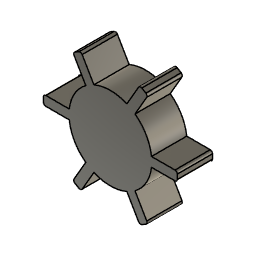
Waterwheel_6 (Autodesk Fusion 360 design; units mm, degrees)
Autodesk Fusion 360 part; units mm, degrees
sketch "スケッチ1" plane through (0, 0, 0) normal (0, 1, 0) x (-1, 0, 0)
  line L0 (-1750, 200) -> (-2750, 200)
  line L1 (-2850, 100) -> (-2850, -100)
  line L2 (-2750, -200) -> (-1750, -200)
  line L3 (-1750, 200) -> (0, 200) construction
  line L4 (0, 200) -> (0, -200) construction
  line L5 (0, -200) -> (-1750, -200) construction
  arc A0 (-2750, 200) -> (-2850, 100) centre (-2750, 100) ccw
  arc A1 (-2850, -100) -> (-2750, -200) centre (-2750, -100) ccw
  line L6 (-173.2051, 100) -> (173.2051, -100) construction
  arc A2 (-1548.2051, -2281.5699) -> (-1511.6025, -2418.1724) centre (-1461.6025, -2331.5699) ccw
  line L7 (-1201.7949, -2481.5699) -> (-701.7949, -1615.5445)
  line L8 (-1048.2051, -1415.5445) -> (-1548.2051, -2281.5699)
  arc A3 (-1338.3975, -2518.1724) -> (-1201.7949, -2481.5699) centre (-1288.3975, -2431.5699) ccw
  line L9 (-1048.2051, -1415.5445) -> (-173.2051, 100) construction
  line L10 (173.2051, -100) -> (-701.7949, -1615.5445) construction
  line L11 (-1511.6025, -2418.1724) -> (-1338.3975, -2518.1724)
  line L12 (-173.2051, -100) -> (173.2051, 100) construction
  arc A4 (1201.7949, -2481.5699) -> (1338.3975, -2518.1724) centre (1288.3975, -2431.5699) ccw
  line L13 (1548.2051, -2281.5699) -> (1048.2051, -1415.5445)
  line L14 (701.7949, -1615.5445) -> (1201.7949, -2481.5699)
  arc A5 (1511.6025, -2418.1724) -> (1548.2051, -2281.5699) centre (1461.6025, -2331.5699) ccw
  line L15 (701.7949, -1615.5445) -> (-173.2051, -100) construction
  line L16 (173.2051, 100) -> (1048.2051, -1415.5445) construction
  line L17 (1338.3975, -2518.1724) -> (1511.6025, -2418.1724)
  line L18 (0, -200) -> (0, 200) construction
  arc A6 (2750, -200) -> (2850, -100) centre (2750, -100) ccw
  line L19 (2750, 200) -> (1750, 200)
  line L20 (1750, -200) -> (2750, -200)
  arc A7 (2850, 100) -> (2750, 200) centre (2750, 100) ccw
  line L21 (1750, -200) -> (0, -200) construction
  line L22 (0, 200) -> (1750, 200) construction
  line L23 (2850, -100) -> (2850, 100)
  line L24 (173.2051, -100) -> (-173.2051, 100) construction
  arc A8 (1548.2051, 2281.5699) -> (1511.6025, 2418.1724) centre (1461.6025, 2331.5699) ccw
  line L25 (1201.7949, 2481.5699) -> (701.7949, 1615.5445)
  line L26 (1048.2051, 1415.5445) -> (1548.2051, 2281.5699)
  arc A9 (1338.3975, 2518.1724) -> (1201.7949, 2481.5699) centre (1288.3975, 2431.5699) ccw
  line L27 (1048.2051, 1415.5445) -> (173.2051, -100) construction
  line L28 (-173.2051, 100) -> (701.7949, 1615.5445) construction
  line L29 (1511.6025, 2418.1724) -> (1338.3975, 2518.1724)
  line L30 (173.2051, 100) -> (-173.2051, -100) construction
  arc A10 (-1201.7949, 2481.5699) -> (-1338.3975, 2518.1724) centre (-1288.3975, 2431.5699) ccw
  line L31 (-1548.2051, 2281.5699) -> (-1048.2051, 1415.5445)
  line L32 (-701.7949, 1615.5445) -> (-1201.7949, 2481.5699)
  arc A11 (-1511.6025, 2418.1724) -> (-1548.2051, 2281.5699) centre (-1461.6025, 2331.5699) ccw
  line L33 (-701.7949, 1615.5445) -> (173.2051, 100) construction
  line L34 (-173.2051, -100) -> (-1048.2051, 1415.5445) construction
  line L35 (-1338.3975, 2518.1724) -> (-1511.6025, 2418.1724)
  arc A12 (-1048.2051, 1415.5445) -> (-1750, 200) centre (0, 0) ccw
  arc A13 (701.7949, 1615.5445) -> (-701.7949, 1615.5445) centre (0, 0) ccw
  arc A14 (1750, 200) -> (1048.2051, 1415.5445) centre (0, 0) ccw
  arc A15 (1048.2051, -1415.5445) -> (1750, -200) centre (0, 0) ccw
  arc A16 (-1750, -200) -> (-1048.2051, -1415.5445) centre (0, 0) ccw
  arc A17 (-701.7949, -1615.5445) -> (701.7949, -1615.5445) centre (0, 0) ccw
  dimension "d19" = 100
  dimension "d20" = 400
  dimension "d21" = 1000
  dimension "d22" = 1750
  dimension "d24" = 360
  constraint coincident A12.centre A13.centre
  constraint horizontal L0
  constraint vertical L1
  constraint horizontal L2
  constraint parallel L0 L3
  constraint perpendicular L3 L4
  constraint perpendicular L4 L5
  constraint midpoint A12.centre L4
  constraint tangent L1 A0
  constraint tangent L0 A0
  constraint tangent L1 A1
  constraint tangent L2 A1
  constraint equal A0 A1
  constraint concentric A12 A16
  constraint concentric A13 A16
  constraint concentric A14 A16
  constraint concentric A15 A16
  constraint concentric A16 A17
  measures "d19" radius of A0
  measures "d20" distance of L0.end L2.start
  measures "d21" distance of L0.start L0.end
  measures "d22" distance of L0.start L3.end
extrude "押し出し1" add sketch "スケッチ1" along normal blind 1500
